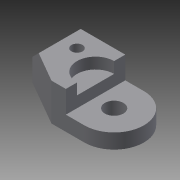
# Autodesk Inventor part: HW 8 Part 2
Saved by Autodesk Inventor 2015 (Build 190159000, 159)
## iProperties
Created: 2016-03-08
Part Number: HW 8 Part 2
Material: Generic
Document SubType Name: Modeling
Designer: Melissa
Density: 1 g/cm^3
Appearance: Default
Author: Melissa
Autodesk Inventor part; units mm, degrees
ref_plane "YZ Plane" through (0, 0, 0) normal (1, 0, 0) x (0, 1, 0)
ref_plane "XZ Plane" through (0, 0, 0) normal (0, 1, 0) x (-1, 0, 0)
ref_plane "XY Plane" through (0, 0, 0) normal (0, 0, 1) x (1, 0, 0)
sketch "Sketch1" plane through (0, 0, 0) normal (0, 0, 1) x (1, 0, 0)
  line L0 (0, 0) -> (0, 38.1)
  line L1 (0, 38.1) -> (25.4, 63.5)
  line L2 (25.4, 63.5) -> (101.6, 63.5)
  line L3 (101.6, 63.5) -> (101.6, 25.4)
  line L4 (101.6, 25.4) -> (133.35, 25.4)
  line L5 (133.35, 25.4) -> (133.35, 0)
  line L6 (133.35, 0) -> (0, 0)
  dimension "d0" = 76.2
  dimension "d1" = 133.35
  dimension "d5" = 45
  dimension "d7" = 31.75
  dimension "d8" = 63.5
  dimension "d9" = 38.1
  constraints: 14 end point, 5 perpendicular, 1 vertical
  measures "d0" distance of L1.end L2.end
  measures "d1" distance of L5.end L0.start
  measures "d5" angle of L2 L1
  measures "d7" distance of L3.end L4.end
  measures "d8" distance between parallel lines of L6 L2
  measures "d9" distance of L2.end L3.end
extrude "Extrusion1" add sketch "Sketch1" along normal blind 101.6
sketch "Sketch2" plane through (101.6, 25.4, 0) normal (0, 1, 0) x (1, 0, 0)
  arc A0 (31.75, -101.6) -> (31.75, 0) centre (31.75, -50.8) ccw
  line L0 (31.75, -101.6) -> (31.75, 0)
  point P0 (-101.6, 0)
  dimension "d12" = 50.8
  constraints: 2 end point, 2 point on circle, 1 centre point, 1 vertical
  measures "d12" radius of A0
extrude "Extrusion2" add sketch "Sketch2" against normal blind 25.4
sketch "Sketch3" plane through (25.4, 63.5, 0) normal (0, 1, 0) x (1, 0, 0)
  line L0 (-25.4, -101.6) -> (51.5897, -101.6)
  line L1 (-25.4, 0) -> (-25.4, -57.15)
  line L2 (-25.4, 0) -> (-25.4, -101.6) projected
  line L3 (-25.4, -57.15) -> (51.5897, -101.6)
  line L4 (-25.4, -57.15) -> (-25.4, -101.6)
  point P0 (76.2, -101.6)
  dimension "d15" = 57.15
  dimension "d16" = 60
  constraints: 8 end point, 1 collinear, 1 horizontal, 1 point on line
  measures "d15" distance of L1.start L1.end
  measures "d16" angle of L3 L2
extrude "Extrusion3" cut sketch "Sketch3" against normal through all
sketch "Sketch4" plane through (25.4, 63.5, 0) normal (0, 1, 0) x (1, 0, 0)
  circle A0 centre (25.4, -31.75) radius 9.525
  line L0 (107.95, 0) -> (-25.4, 0) projected
  line L1 (76.2, 0) -> (76.2, -101.6) projected
  dimension "d19" = 19.05
  dimension "d20" = 31.75
  dimension "d21" = 50.8
  constraints: 1 centre point
  measures "d19" diameter of A0
  measures "d20" distance from line of L0 A0.centre
  measures "d21" distance from line of L1 A0.centre
extrude "Extrusion4" cut sketch "Sketch4" against normal through all
sketch "Sketch6" plane through (101.6, 25.4, 101.6) normal (0, 1, 0) x (1, 0, 0)
  arc A0 (31.75, 0) -> (31.75, 101.6) centre (31.75, 50.8) ccw projected
  circle A1 centre (31.75, 50.8) radius 15.875
  point P0 (-101.6, 101.6)
  dimension "d25" = 31.75
  constraints: 1 centre point, 1 coincident
  measures "d25" diameter of A1
extrude "Extrusion5" cut sketch "Sketch6" against normal through all
sketch "Sketch7" plane through (25.4, 63.5, 0) normal (0, 1, 0) x (1, 0, 0)
  line L0 (76.2, 0) -> (76.2, -101.6) projected
  arc A0 (76.2, -19.05) -> (76.2, -82.55) centre (76.2, -50.8) ccw
  line L1 (76.2, -82.55) -> (76.2, -19.05)
  point P0 (-25.4, 0)
  dimension "d28" = 63.5
  constraints: 2 end point, 2 point on circle, 2 point on line, 1 centre point, 1 midpoint
  measures "d28" diameter of A0
extrude "Extrusion6" cut sketch "Sketch7" against normal blind 19.05
body "Solid1"
